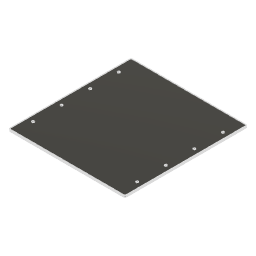
deck_panel_front (Autodesk Fusion 360 design; units mm, degrees)
Autodesk Fusion 360 part; units mm, degrees
sketch "Sketch1" plane through (0, 0, 0) normal (0, 0, 1) x (1, 0, 0)
  line L0 (90, -6.35) -> (90, -206.35)
  line L1 (280, -206.35) -> (280, -6.35)
  line L2 (90, -206.35) -> (280, -206.35)
  line L3 (280, -6.35) -> (90, -6.35)
  line L4 (100, -6.35) -> (100, -206.35) construction
  line L5 (185, -6.35) -> (185, -206.35)
  circle A0 centre (100, -176.35) radius 1.7
  circle A1 centre (100, -129.6833) radius 1.7
  circle A2 centre (100, -83.0167) radius 1.7
  circle A3 centre (100, -36.35) radius 1.7
  circle A4 centre (270, -176.35) radius 1.7
  circle A5 centre (270, -129.6833) radius 1.7
  circle A6 centre (270, -83.0167) radius 1.7
  circle A7 centre (270, -36.35) radius 1.7
  circle A8 centre (93, -203.35) radius 3
  circle A9 centre (93, -9.35) radius 3
  circle A10 centre (277, -9.35) radius 3
  circle A11 centre (277, -203.35) radius 3
  dimension "d3694" = 200
  dimension "d3695" = 90
  dimension "d3696" = 6.35
  dimension "d3697" = 190
  dimension "d3698" = 100
  dimension "d3699" = 3.4
  dimension "d3700" = 30
  dimension "d3701" = 30
  dimension "d3702" = 46.6667
  dimension "d3703" = 46.6667
  dimension "d3706" = 6
  constraint coincident L0.end L2.start
  constraint coincident L1.start L2.end
  constraint coincident L1.end L3.start
  constraint coincident L0.start L3.end
  constraint vertical L0
  constraint horizontal L3
  constraint vertical L1
  constraint horizontal L2
  constraint coincident L3 L4.start
  constraint coincident L2 L4.end
  constraint vertical L4
  constraint midpoint L3 L5.start
  constraint midpoint L2 L5.end
  constraint coincident L4 A0.centre
  constraint coincident L4 A1.centre
  constraint coincident L4 A2.centre
  constraint coincident L4 A3.centre
  constraint equal A2 A3
  constraint equal A1 A2
  constraint equal A0 A1
  constraint symmetric L5 A0 A4
  constraint symmetric L5 A1 A5
  constraint symmetric L5 A2 A6
  constraint symmetric L5 A3 A7
  constraint tangent L2 A8
  constraint tangent L0 A8
  constraint equal A8 A9
  constraint tangent L0 A9
  constraint tangent L3 A9
  constraint symmetric L5 A8 A11
  constraint symmetric L5 A9 A10
  measures "d3694" distance of L0.start L0.end
  measures "d3695" distance of origin L0
  measures "d3696" distance of origin L3
  measures "d3697" distance of L0.end L1.start
  measures "d3698" distance of origin L4
  measures "d3699" diameter of A0
  measures "d3700" distance of L2 A0.centre
  measures "d3701" distance of L3 A3.centre
  measures "d3702" distance of A0.centre A1.centre
  measures "d3703" distance of A2.centre A3.centre
  measures "d3706" diameter of A8
extrude "Extrude1" add sketch "Sketch1" along normal blind 3 contours L0 L2 L3 L5 A8 A9 | A9 | A8 | L1 L2 L3 L5 A10 A11 | A10 | A11
sketch "DXF" plane through (0, 0, 3) normal (0, 0, 1) x (-1, 0, 0)
  circle A0 centre (-270, 176.35) radius 1.7
  circle A1 centre (-100, 36.35) radius 1.7
  circle A2 centre (-270, 36.35) radius 1.7
  circle A3 centre (-100, 83.0167) radius 1.7
  circle A4 centre (-100, 176.35) radius 1.7
  circle A5 centre (-270, 83.0167) radius 1.7
  circle A6 centre (-100, 129.6833) radius 1.7
  circle A7 centre (-270, 129.6833) radius 1.7
  line L0 (-93, 206.35) -> (-277, 206.35)
  arc A8 (-277, 206.35) -> (-280, 203.35) centre (-277, 203.35) ccw
  line L1 (-280, 203.35) -> (-280, 9.35)
  arc A9 (-280, 9.35) -> (-277, 6.35) centre (-277, 9.35) ccw
  line L2 (-277, 6.35) -> (-93, 6.35)
  arc A10 (-93, 6.35) -> (-90, 9.35) centre (-93, 9.35) ccw
  line L3 (-90, 9.35) -> (-90, 203.35)
  arc A11 (-90, 203.35) -> (-93, 206.35) centre (-93, 203.35) ccw
chamfer "Chamfer1" distance 0.4 angle 45 16 edges at (280, -106.35, 0) (279.1213, -7.2287, 0) (185, -6.35, 0) (90.8787, -7.2287, 0) (90, -106.35, 0) (90.8787, -205.4713, 0) (185, -206.35, 0) (279.1213, -205.4713, 0) (280, -106.35, 3) (279.1213, -7.2287, 3) (185, -6.35, 3) (90.8787, -7.2287, 3) (90, -106.35, 3) (90.8787, -205.4713, 3) (185, -206.35, 3) (279.1213, -205.4713, 3)
equation "d3694 = 204 mm - 3 mm - 1 mm"
equation "d3696 = 5.35 mm + 1 mm"
equation "d3698 = 85 mm + 15 mm"
equation "d3702 = ( d3694 - ( d3700 * 2 ) ) / 3"
equation "d3703 = d3702"
